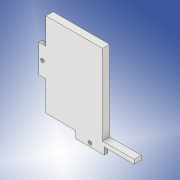
# Autodesk Inventor part: TC004
Saved by Autodesk Inventor 2017 SP1 (Build 210196100, 196)
## iProperties
Created: 2017-08-15
Part Number: TC004
Material: ABS Plastic
Document SubType Name: Modeling
Designer: Zach
Density: 1.06 g/cm^3
Appearance: CR White
Author: Zach
Autodesk Inventor part; units mm, degrees
ref_plane "YZ Plane" through (0, 0, 0) normal (1, 0, 0) x (0, 1, 0)
ref_plane "XZ Plane" through (0, 0, 0) normal (0, 1, 0) x (-1, 0, 0)
ref_plane "XY Plane" through (0, 0, 0) normal (0, 0, 1) x (1, 0, 0)
sketch "Sketch1" plane through (0, 0, 0) normal (0, 0, 1) x (1, 0, 0)
  line L0 (0, 0) -> (124, 0)
  line L1 (124, 0) -> (124, 124)
  line L2 (124, 124) -> (0, 124)
  line L3 (0, 124) -> (0, 0)
  dimension "d0" = 124
  dimension "d1" = 124
  constraints: 8 end point, 2 parallel, 1 horizontal, 1 perpendicular
  measures "d0" distance of L2.end L1.end
  measures "d1" distance of L1.end L0.end
extrude "Extrusion1" add sketch "Sketch1" along normal blind 10
sketch "Sketch2" plane through (0, 0, 10) normal (0, 0, 1) x (1, 0, 0)
  line L0 (124, 0) -> (124, 124) projected
  line L1 (124, 124) -> (79.5, 124)
  line L2 (79.5, 124) -> (79.5, 6)
  line L3 (79.5, 6) -> (124, 6)
  line L4 (124, 6) -> (124, 124)
  point P0 (0, 0)
  dimension "d4" = 44.5
  dimension "d5" = 118
  constraints: 8 end point, 2 parallel, 1 horizontal, 1 perpendicular
  measures "d4" distance of L3.end L2.end
  measures "d5" distance of L1.end L2.end
extrude "Extrusion2" cut sketch "Sketch2" against normal through all
sketch "Sketch3" plane through (0, 0, 10) normal (0, 0, 1) x (1, 0, 0)
  line L0 (0, 124) -> (0, 0) projected
  line L1 (0, 82) -> (-10, 82)
  line L2 (-10, 82) -> (-10, 42)
  line L3 (-10, 42) -> (0, 42)
  line L4 (0, 42) -> (0, 82)
  circle A0 centre (-5, 62) radius 2.5
  line L5 (0, 0) -> (124, 0) projected
  line L6 (42, 0) -> (82, 0)
  line L7 (82, 0) -> (82, -10)
  line L8 (82, -10) -> (42, -10)
  line L9 (42, -10) -> (42, 0)
  circle A1 centre (62, -5) radius 2.5
  point P0 (-10, 62)
  point P1 (0, 62)
  point P2 (-5, 82)
  point P3 (62, -10)
  point P4 (62, 0)
  point P5 (62, 0)
  point P6 (42, -5)
  dimension "d8" = 10
  dimension "d9" = 40
  dimension "d10" = 5
  dimension "d11" = 40
  dimension "d12" = 10
  dimension "d13" = 5
  constraints: 16 end point, 7 midpoint, 4 parallel, 3 horizontal alignment, 2 centre point, 2 horizontal, 2 perpendicular, 2 point on line, 2 vertical alignment, 1 coincident
  measures "d8" distance of L3.end L2.end
  measures "d9" distance of L2.end L1.end
  measures "d10" diameter of A0
  measures "d11" distance of L7.end L8.end
  measures "d12" distance of L6.end L7.end
  measures "d13" diameter of A1
extrude "Extrusion3" add sketch "Sketch3" against normal blind 5
sketch "Sketch5" plane through (0, 0, 10) normal (0, 0, 1) x (1, 0, 0)
  line L0 (0, 124) -> (0, 82) projected
  line L1 (0, 124) -> (79.5, 124)
  line L2 (79.5, 124) -> (79.5, 119)
  line L3 (79.5, 119) -> (0, 119)
  line L4 (0, 119) -> (0, 124)
  line L5 (79.5, 6) -> (79.5, 124) projected
  point P0 (0, 0)
  dimension "d19" = 5
  constraints: 8 end point, 2 parallel, 1 horizontal, 1 perpendicular, 1 point on line
  measures "d19" distance of L1.end L2.end
extrude "Extrusion5" cut sketch "Sketch5" against normal through all
body "Solid1"
